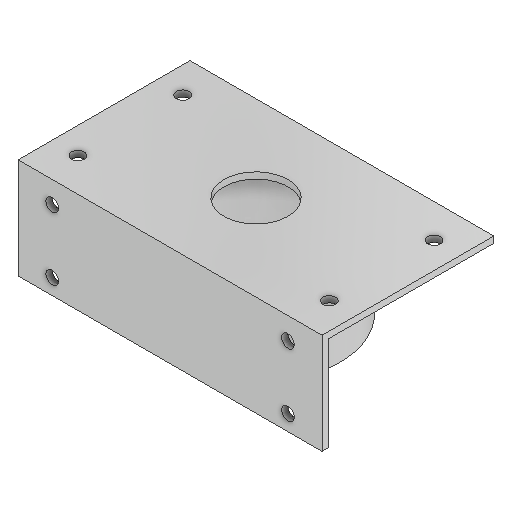
# Autodesk Inventor part: WheelHolder
Saved by Autodesk Inventor 2022 (Build 260153000, 153)
## iProperties
Created: 2024-07-10
Part Number: WheelHolder
Material: Aluminum 6061-AHC
Document SubType Name: Modeling
Designer: LaptopJR
Density: 2.7 g/cm^3
Appearance: Aluminum - Dark
Author: LaptopJR
Autodesk Inventor part; units mm, degrees
ref_plane "YZ Plane" through (0, 0, 0) normal (1, 0, 0) x (0, 1, 0)
ref_plane "XZ Plane" through (0, 0, 0) normal (0, 1, 0) x (-1, 0, 0)
ref_plane "XY Plane" through (0, 0, 0) normal (0, 0, 1) x (1, 0, 0)
sketch "Sketch1" plane through (0, 0, 0) normal (0, 1, 0) x (-1, 0, 0)
  circle A0 centre (0, 0) radius 15.25
  circle A1 centre (0, 0) radius 32.5 construction
  line L0 (0, 0) -> (0, -32.5) construction
  line L1 (0, 0) -> (-22.981, -22.981) construction
  circle A2 centre (-22.981, -22.981) radius 3.05 construction
  circle A3 centre (22.981, -22.981) radius 3.05 construction
  circle A4 centre (22.981, 22.981) radius 3.05 construction
  circle A5 centre (-22.981, 22.981) radius 3.05 construction
  circle A6 centre (0, 0) radius 40
  circle A7 centre (22.981, -22.981) radius 5 construction
  dimension "d0" = 30.5
  dimension "d1" = 6.1
  dimension "d3" = 45
  dimension "d4" = 65
  dimension "d7" = 360
  dimension "d9" = 80
  dimension "d10" = 10
  constraints: 8 centre point, 5 coincident, 4 end point, 2 point on circle, 1 vertical, 9 other
  measures "d0" diameter of A0
  measures "d1" diameter of A2
  measures "d3" angle of L1 L0
  measures "d4" diameter of A1
  measures "d9" diameter of A6
  measures "d10" diameter of A7
extrude "Extrusion1" add sketch "Sketch1" along normal blind 3
sketch "Sketch2" plane through (0, 0, 0) normal (0, -1, 0) x (1, 0, 0)
  circle A0 centre (0, 0) radius 40 projected
  circle A1 centre (0, 0) radius 37
  dimension "d13" = 3
  constraints: 1 centre point, 1 coincident
  measures "d13" radial gap between concentric circles of A0 A1
extrude "Extrusion2" add sketch "Sketch2" along normal blind 45
sketch "Sketch3" plane through (0, 3, 0) normal (0, 1, 0) x (1, 0, 0)
  line L0 (-72.5, -41) -> (72.5, -41)
  line L1 (72.5, -41) -> (72.5, 41)
  line L2 (72.5, 41) -> (-72.5, 41)
  line L3 (-72.5, 41) -> (-72.5, -41)
  line L4 (-72.5, -41) -> (72.5, 41) construction
  line L5 (72.5, -41) -> (-72.5, 41) construction
  circle A0 centre (0, 0) radius 40 projected
  circle A1 centre (0, 0) radius 15.25 projected
  line L6 (-60, -25) -> (60, -25) construction
  line L7 (60, -25) -> (60, 25) construction
  line L8 (60, 25) -> (-60, 25) construction
  line L9 (-60, 25) -> (-60, -25) construction
  line L10 (-60, -25) -> (60, 25) construction
  line L11 (60, -25) -> (-60, 25) construction
  circle A2 centre (-60, 25) radius 3.05
  circle A3 centre (-60, -25) radius 3.05
  circle A4 centre (60, 25) radius 3.05
  circle A5 centre (60, -25) radius 3.05
  dimension "d16" = 145
  dimension "d17" = 82
  dimension "d18" = 120
  dimension "d19" = 50
  dimension "d20" = 6.1
  constraints: 24 end point, 4 centre point, 4 coincident, 4 midpoint, 4 parallel, 3 equal radius, 2 horizontal, 2 perpendicular
  measures "d16" distance of L2.end L1.end
  measures "d17" distance of L1.end L0.end
  measures "d18" distance of L8.end L7.end
  measures "d19" distance of L7.end L6.end
  measures "d20" diameter of A2
extrude "Extrusion3" add sketch "Sketch3" against normal blind 3 contours L3 L2 L1 L0
sketch "Sketch4" plane through (-72.5, 3, 41) normal (0, 0, 1) x (1, 0, 0)
  line L0 (32.5, -3) -> (112.5, -3) projected
  line L1 (32.5, -48) -> (112.5, -48) projected
  line L2 (0, 0) -> (145, 0) projected
  line L3 (0, 0) -> (0, -3) projected
  line L4 (145, -3) -> (0, -3) projected
  line L5 (145, 0) -> (145, -3) projected
  line L6 (0, 0) -> (0, -3) projected
  line L7 (32.5, -48) -> (112.5, -48) projected
  line L8 (0, -3) -> (32.5, -3)
  line L9 (32.5, -3) -> (32.5, -48)
  line L10 (32.5, -48) -> (0, -48)
  line L11 (0, -48) -> (0, -3)
  line L12 (112.5, -48) -> (145, -48)
  line L13 (145, -48) -> (145, -3)
  line L14 (145, -3) -> (112.5, -3)
  line L15 (112.5, -3) -> (112.5, -48)
  line L16 (16.25, -48) -> (16.25, -3) construction
  line L17 (145, -3) -> (0, -3) projected
  line L18 (128.75, -48) -> (128.75, -3) construction
  circle A0 centre (16.25, -40.5) radius 3.05
  line L19 (16.25, -40.5) -> (128.75, -40.5) construction
  line L20 (128.75, -40.5) -> (128.75, -10.5) construction
  line L21 (128.75, -10.5) -> (16.25, -10.5) construction
  line L22 (16.25, -10.5) -> (16.25, -40.5) construction
  circle A1 centre (16.25, -10.5) radius 3.05
  circle A2 centre (128.75, -10.5) radius 3.05
  circle A3 centre (128.75, -40.5) radius 3.05
  point P0 (72.5, -3)
  dimension "d23" = 30
  dimension "d24" = 7.5
  dimension "d25" = 6.1
  constraints: 28 end point, 6 parallel, 5 perpendicular, 4 centre point, 3 coincident, 3 equal radius, 3 horizontal, 2 midpoint, 2 point on line, 3 other
  measures "d23" distance between parallel lines of L19 L21
  measures "d24" distance between parallel lines of L10 L19
  measures "d25" diameter of A1
extrude "Extrusion4" add sketch "Sketch4" against normal blind 3 contours L9 L10 L11 L4 | L0 L15 L1 L9 | L4 L13 L12 L15
body "Solid1"
